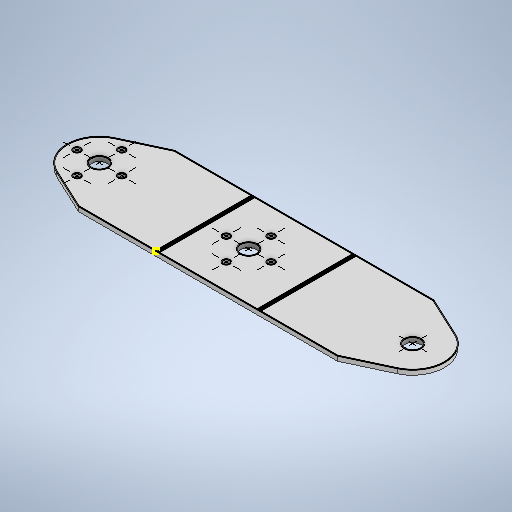
# Autodesk Inventor part: CAM_axis_1_top_frame
Saved by Autodesk Inventor 2025.2 (Build 292293000, 293)
## iProperties
Created: 2025-08-09
Part Number: CAM_axis_1_top_frame
Material: Generic
Document SubType Name: Modeling
Designer: User
Density: 1 g/cm^3
Appearance: Default
Author: User
Autodesk Inventor part; units mm, degrees
ref_plane "YZ Plane" through (0, 0, 0) normal (1, 0, 0) x (0, 1, 0)
ref_plane "XZ Plane" through (0, 0, 0) normal (0, 1, 0) x (-1, 0, 0)
ref_plane "XY Plane" through (0, 0, 0) normal (0, 0, 1) x (1, 0, 0)
sketch "Sketch1" plane through (0, 0, 0) normal (0, 1, 0) x (-1, 0, 0)
  line L0 (-0.4496, -30) -> (-0.4496, 0)
  line L1 (-32.1589, 0) -> (-32.1589, -30)
  circle A0 centre (-65.2986, -15) radius 2.55
  circle A1 centre (32.69, -15) radius 2.6
  circle A2 centre (-7.0193, -15) radius 1.05
  circle A3 centre (-14.0193, -8) radius 1.05
  circle A4 centre (-14.0193, -22) radius 1.05
  circle A5 centre (-21.0193, -15) radius 1.05
  circle A6 centre (-14.0193, -15) radius 2.6
  circle A7 centre (25.69, -15) radius 1.05
  circle A8 centre (32.69, -8) radius 1.05
  circle A9 centre (32.69, -22) radius 1.05
  circle A10 centre (39.69, -15) radius 1.05
  line L2 (36.9177, -5.9376) -> (24.19, 0)
  line L3 (-56.7986, 0) -> (-69.5263, -5.9376)
  arc A11 (36.9177, -24.0624) -> (36.9177, -5.9376) centre (32.69, -15) ccw
  line L4 (24.19, -30) -> (36.9177, -24.0624)
  line L5 (-69.5263, -24.0624) -> (-56.7986, -30)
  arc A12 (-69.5263, -5.9376) -> (-69.5263, -24.0624) centre (-65.2986, -15) ccw
  line L6 (-56.7986, 0) -> (24.19, 0)
  line L7 (24.19, -30) -> (-56.7986, -30)
  line L8 (-32.6086, -30) -> (-32.6086, 0)
  line L9 (-31.7093, 0) -> (-31.7093, -30)
  line L10 (-0.8993, -30) -> (-0.8993, 0)
  line L11 (0, 0) -> (0, -30)
  point P0 (0, 0)
  constraints: 24 end point, 13 centre point, 12 point on line, 9 equal radius, 7 parallel, 6 vertical, 4 point on circle, 4 tangent, 2 horizontal, 2 perpendicular, 49 other
extrude "Extrusion1" add sketch "Sketch1" against normal blind 1.5
body "Solid1"
